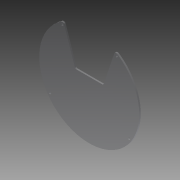
# Autodesk Inventor part: Top Plate
Saved by Autodesk Inventor 2015 (Build 190159000, 159)
## iProperties
Created: 2016-09-20
Part Number: Top Plate
Material: Generic
Document SubType Name: Modeling
Designer: James Yelland
Density: 1 g/cm^3
Appearance: Default
Author: James Yelland
Autodesk Inventor part; units mm, degrees
ref_plane "YZ Plane" through (0, 0, 0) normal (1, 0, 0) x (0, 1, 0)
ref_plane "XZ Plane" through (0, 0, 0) normal (0, 1, 0) x (-1, 0, 0)
ref_plane "XY Plane" through (0, 0, 0) normal (0, 0, 1) x (1, 0, 0)
sketch "Sketch1" plane through (0, 0, 0) normal (0, 1, 0) x (-1, 0, 0)
  circle A0 centre (-54.4898, 77.8194) radius 1.6
  circle A1 centre (54.4898, 77.8194) radius 1.6
  circle A2 centre (-78.9896, -52.7792) radius 1.6
  circle A3 centre (78.9896, -52.7792) radius 1.6
  line L0 (0, 15) -> (25.841, 15)
  line L1 (0, 15) -> (-25.841, 15)
  line L2 (-54.8544, 83) -> (-52.9353, 83)
  line L3 (-50.0906, 80.9528) -> (-28.6857, 17.0472)
  line L4 (54.8544, 83) -> (52.9353, 83)
  line L5 (50.0906, 80.9528) -> (28.6857, 17.0472)
  arc A4 (-56.5509, 82.4742) -> (56.5509, 82.4742) centre (0, 0) ccw
  arc A5 (56.5509, 82.4742) -> (54.8544, 83) centre (54.8544, 80) ccw
  arc A6 (52.9353, 83) -> (50.0906, 80.9528) centre (52.9353, 80) ccw
  arc A7 (25.841, 15) -> (28.6857, 17.0472) centre (25.841, 18) ccw
  arc A8 (-28.6857, 17.0472) -> (-25.841, 15) centre (-25.841, 18) ccw
  arc A9 (-50.0906, 80.9528) -> (-52.9353, 83) centre (-52.9353, 80) ccw
  arc A10 (-54.8544, 83) -> (-56.5509, 82.4742) centre (-54.8544, 80) ccw
  point P0 (-54.3117, 78)
  point P1 (54.3117, 78)
  point P2 (55.7763, 83)
  point P3 (-55.7763, 83)
  point P4 (28, 15)
  point P5 (-28, 15)
  point P6 (-50.7763, 83)
  point P7 (50.7763, 83)
  dimension "d11" = 3.2
  dimension "d12" = 3.2
  dimension "d13" = 3.2
  dimension "d14" = 3.2
  dimension "d34" = 28
  dimension "d35" = 28
  dimension "d36" = 5
  dimension "d37" = 5
  dimension "d38" = 3
  constraints: 16 point on circle, 12 end point, 12 tangent, 11 centre point, 10 point on line, 5 equal radius, 2 horizontal
  measures "d11" diameter of A0
  measures "d12" diameter of A1
  measures "d13" diameter of A2
  measures "d14" diameter of A3
  measures "d34" distance of L0.start point (28, 15)
  measures "d35" distance of L0.start point (-28, 15)
  measures "d36" distance of point (-55.776, 83) point (-50.776, 83)
  measures "d37" distance of point (55.776, 83) point (50.776, 83)
  measures "d38" radius of A5
extrude "Extrusion1" add sketch "Sketch1" along normal blind 3
body "Solid1"
